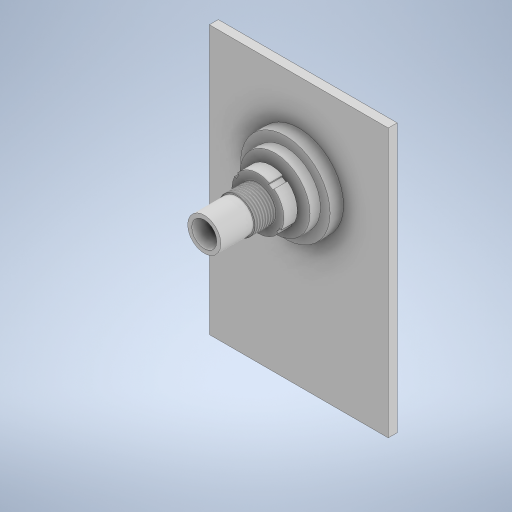
# Autodesk Inventor part: lathe_spindle_end
Saved by Autodesk Inventor 2023 (Build 270158000, 158)
## iProperties
Created: 2023-10-19
Part Number: lathe_spindle_end
Material: Generic
Document SubType Name: Modeling
Designer: mark
Density: 1 g/cm^3
Appearance: Default
Author: mark
Autodesk Inventor part; units mm, degrees
ref_plane "YZ Plane" through (0, 0, 0) normal (1, 0, 0) x (0, 1, 0)
ref_plane "XZ Plane" through (0, 0, 0) normal (0, 1, 0) x (-1, 0, 0)
ref_plane "XY Plane" through (0, 0, 0) normal (0, 0, 1) x (1, 0, 0)
sketch "Sketch1" plane through (0, 0, 0) normal (0, 0, 1) x (1, 0, 0)
  line L0 (-99.623, 141.7467) -> (100.377, 141.7467)
  line L1 (100.377, 141.7467) -> (100.377, -158.2533)
  line L2 (100.377, -158.2533) -> (-99.623, -158.2533)
  line L3 (-99.623, -158.2533) -> (-99.623, 141.7467)
  point P0 (0, 0)
  dimension "d0" = 200
  dimension "d1" = 300
  constraints: 8 end point, 2 parallel, 1 horizontal, 1 perpendicular
  measures "d0" distance of L0.start L0.end
  measures "d1" distance of L2.end L0.start
extrude "Extrusion1" add sketch "Sketch1" along normal blind 10
sketch "Sketch2" plane through (0, 0, 10) normal (0, 0, 1) x (1, 0, 0)
  circle A0 centre (0.377, 41.7467) radius 50
  line L0 (100.377, 141.7467) -> (-99.623, 141.7467) projected
  line L1 (100.377, -158.2533) -> (100.377, 141.7467) projected
  point P0 (0, 0)
  dimension "d4" = 100
  dimension "d5" = 100
  dimension "d6" = 100
  constraints: 1 centre point
  measures "d4" diameter of A0
  measures "d5" distance from line of L0 A0.centre
  measures "d6" distance from line of L1 A0.centre
extrude "Extrusion2" add sketch "Sketch2" along normal blind 15
sketch "Sketch3" plane through (0.377, 41.7467, 25) normal (0, 0, 1) x (1, 0, 0)
  circle A0 centre (0, 0) radius 39.25
  point P0 (-0.377, -41.7467)
  dimension "d9" = 78.5
  constraints: 1 centre point
  measures "d9" diameter of A0
extrude "Extrusion3" add sketch "Sketch3" along normal blind 11.7
sketch "Sketch4" plane through (0.377, 41.7467, 36.7) normal (0, 0, 1) x (1, 0, 0)
  circle A0 centre (0, 0) radius 18.555
  point P0 (-0.377, -41.7467)
  dimension "d12" = 37.11
  constraints: 1 centre point
  measures "d12" diameter of A0
extrude "Extrusion4" add sketch "Sketch4" along normal blind 79
ref_plane "Work Plane1" through (0.377, 41.7467, 40.7) normal (0, 0, 1) x (1, 0, 0)
sketch "Sketch5" plane through (0.377, 41.7467, 40.7) normal (0, 0, 1) x (1, 0, 0)
  circle A0 centre (0, 0) radius 18.555 projected
  circle A1 centre (0, 0) radius 29.09
  circle A2 centre (0, 0) radius 26.79
  line L0 (0, 0) -> (12.9512, 26.0479)
  line L1 (0, 0) -> (18.044, 22.8176)
  line L2 (0, 0) -> (-26.0479, 12.9512)
  line L3 (0, 0) -> (-22.8176, 18.044)
  line L4 (0, 0) -> (-12.9512, -26.0479)
  line L5 (0, 0) -> (-18.044, -22.8176)
  line L6 (0, 0) -> (26.0479, -12.9512)
  line L7 (0, 0) -> (22.8176, -18.044)
  point P0 (-0.377, -41.7467)
  point P1 (-23.9885, 11.9272)
  point P2 (-18.044, -22.8176)
  point P3 (-16.6174, -21.0135)
  point P4 (-11.9272, -23.9885)
  point P5 (22.8176, -18.044)
  point P6 (21.0135, -16.6174)
  point P7 (23.9885, -11.9272)
  point P8 (26.0479, -12.9512)
  point P9 (16.6174, 21.0135)
  point P10 (11.9272, 23.9885)
  point P11 (-21.0135, 16.6174)
  dimension "d16" = 58.18
  dimension "d19" = 53.58
  dimension "d20" = 11.9
  dimension "d23" = 360
  constraints: 16 end point, 2 centre point, 2 coincident, 2 point on circle, 21 other
  measures "d16" diameter of A1
  measures "d19" diameter of A2
  measures "d20" angle of L1 L0
extrude "Extrusion5" add sketch "Sketch5" along normal blind 15 contours A0 L1 A2 L6 | A0 L0 A2 L1 | L6 A2 L7 A0 | A0 L3 A2 L0 | L1 A1 L6 A2 | L7 A2 L4 A0 | A0 L2 A2 L3 | A2 L3 A1 L0 | A0 L5 A2 L2 | L4 A2 L5 A0 | L7 A1 L4 A2 | A2 L5 A1 L2
sketch "Sketch6" plane through (0.377, 41.7467, 115.7) normal (0, 0, 1) x (1, 0, 0)
  circle A0 centre (0, 0) radius 14
  point P0 (-0.377, -41.7467)
  dimension "d25" = 28
  constraints: 1 centre point
  measures "d25" diameter of A0
extrude "Extrusion6" cut sketch "Sketch6" against normal through all
sketch "Sketch7" plane through (0.377, 41.7467, 55.7) normal (0, 0, 1) x (1, 0, 0)
  circle A0 centre (0, 0) radius 14
  circle A1 centre (0, 0) radius 20
  point P0 (-0.377, -41.7467)
  dimension "d28" = 40
  constraints: 2 centre point, 1 coincident
  measures "d28" diameter of A1
extrude "Extrusion7" add sketch "Sketch7" along normal blind 23.5
thread "Thread1" size "M40x3" class "6g" standard "ANSI Metric M Profile" full length
body "Solid1"
